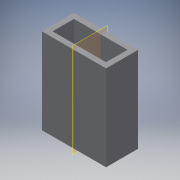
# Autodesk Inventor part: magnetHolder
Saved by Autodesk Inventor 2018.2 (Build 222227000, 227)
## iProperties
Created: 2018-03-20
Part Number: magnetHolder
Material: Aluminum 6061
Document SubType Name: Modeling
Designer: steele
Density: 2.7 g/cm^3
Appearance: Canary
Author: steele
Autodesk Inventor part; units mm, degrees
ref_plane "XZ Plane" through (0, 0, 0) normal (0, 1, 0) x (-1, 0, 0)
ref_plane "XY Plane" through (0, 0, 0) normal (0, 0, 1) x (1, 0, 0)
sketch "Sketch1" plane through (0, 0, 0) normal (0, 0, 1) x (1, 0, 0)
  line L0 (-19.05, -25.4) -> (19.05, -25.4)
  line L1 (19.05, -25.4) -> (19.05, 25.4)
  line L2 (19.05, 25.4) -> (-19.05, 25.4)
  line L3 (-19.05, 25.4) -> (-19.05, -25.4)
  line L4 (-19.05, -25.4) -> (19.05, 25.4) construction
  line L5 (19.05, -25.4) -> (-19.05, 25.4) construction
  point P0 (0, 0)
  dimension "d0" = 38.1
  dimension "d1" = 50.8
  constraints: 12 end point, 2 midpoint, 2 parallel, 1 horizontal, 1 perpendicular
  measures "d0" distance of L1.end L2.end
  measures "d1" distance of L2.end L0.start
extrude "Extrusion1" add sketch "Sketch1" along normal mid plane 19.05
sketch "Sketch2" plane through (-19.05, 25.4, 9.525) normal (0, 1, 0) x (1, 0, 0)
  line L0 (34.925, 3.175) -> (34.925, 15.875)
  line L1 (34.925, 15.875) -> (3.175, 15.875)
  line L2 (3.175, 15.875) -> (3.175, 3.175)
  line L3 (3.175, 3.175) -> (34.925, 3.175)
  line L4 (34.925, 3.175) -> (3.175, 15.875) construction
  line L5 (34.925, 15.875) -> (3.175, 3.175) construction
  line L6 (0, 19.05) -> (38.1, 19.05) projected
  line L7 (0, 19.05) -> (0, 0) projected
  point P0 (19.05, 9.525)
  dimension "d4" = 3.175
  dimension "d5" = 3.175
  constraints: 12 end point, 2 midpoint, 2 parallel, 1 perpendicular, 1 vertical
  measures "d4" distance between parallel lines of L6 L1
  measures "d5" distance between parallel lines of L7 L2
extrude "Extrusion2" cut sketch "Sketch2" against normal through all
body "Solid1"
